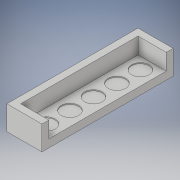
# Autodesk Inventor part: conteneur-boues
Saved by Autodesk Inventor 2019 (Build 230136000, 136)
## iProperties
Created: 2020-02-15
Part Number: conteneur-boues
Material: Generic
Document SubType Name: Modeling
Designer: franc
Density: 1 g/cm^3
Appearance: Default
Author: franc
Autodesk Inventor part; units mm, degrees
ref_plane "YZ Plane" through (0, 0, 0) normal (1, 0, 0) x (0, 1, 0)
ref_plane "XZ Plane" through (0, 0, 0) normal (0, 1, 0) x (-1, 0, 0)
ref_plane "XY Plane" through (0, 0, 0) normal (0, 0, 1) x (1, 0, 0)
sketch "Esquisse1" plane through (0, 0, 0) normal (0, 1, 0) x (-1, 0, 0)
  line L0 (56.6857, 276.3714) -> (-55.3143, 276.3714)
  line L1 (-55.3143, 276.3714) -> (-55.3143, -142.6286)
  line L2 (-55.3143, -142.6286) -> (56.6857, -142.6286)
  line L3 (56.6857, -142.6286) -> (56.6857, 276.3714)
  point P0 (0, 0)
  dimension "d0" = 112
  dimension "d1" = 419
  constraints: 8 end point, 2 parallel, 1 horizontal, 1 perpendicular
  measures "d0" distance of L1.end L2.end
  measures "d1" distance of L2.end L0.start
extrude "Extrusion1" add sketch "Esquisse1" along normal blind 22
sketch "Esquisse2" plane through (0, 22, 0) normal (0, 1, 0) x (1, 0, 0)
  line L0 (-56.6857, 142.6286) -> (-56.6857, -276.3714) projected
  line L1 (55.3143, -276.3714) -> (55.3143, 142.6286) projected
  line L2 (-56.6857, -276.3714) -> (55.3143, -276.3714)
  line L3 (55.3143, -276.3714) -> (55.3143, -254.3714)
  line L4 (55.3143, -254.3714) -> (-56.6857, -254.3714)
  line L5 (-56.6857, -254.3714) -> (-56.6857, -276.3714)
  line L6 (55.3143, 142.6286) -> (-56.6857, 142.6286) projected
  line L7 (-56.6857, 142.6286) -> (55.3143, 142.6286)
  line L8 (55.3143, 142.6286) -> (55.3143, 120.6286)
  line L9 (55.3143, 120.6286) -> (-56.6857, 120.6286)
  line L10 (-56.6857, 120.6286) -> (-56.6857, 142.6286)
  line L11 (-56.6857, -254.3714) -> (-34.6857, -254.3714)
  line L12 (-34.6857, -254.3714) -> (-34.6857, 120.6286)
  line L13 (-34.6857, 120.6286) -> (-56.6857, 120.6286)
  line L14 (-56.6857, 120.6286) -> (-56.6857, -254.3714)
  point P0 (0, 0)
  dimension "d4" = 22
  dimension "d5" = 22
  dimension "d6" = 22
  constraints: 24 end point, 6 parallel, 3 horizontal, 3 perpendicular, 3 point on line
  measures "d4" distance between parallel lines of L2 L4
  measures "d5" distance between parallel lines of L0 L12
  measures "d6" distance between parallel lines of L6 L9
extrude "Extrusion2" add sketch "Esquisse2" along normal blind 55 contours L6 L1 L9 L0 | L9 L12 L4 L0 | L4 L1 L2 L0
sketch "Esquisse3" plane through (0, 22, 0) normal (0, 1, 0) x (1, 0, 0)
  line L0 (-34.6857, 120.6286) -> (-34.6857, -254.3714) projected
  line L1 (-34.6857, 120.6286) -> (55.3143, 120.6286) projected
  line L2 (-34.6857, -254.3714) -> (55.3143, -254.3714)
  line L3 (55.3143, -254.3714) -> (55.3143, 120.6286)
  line L4 (55.3143, 120.6286) -> (-34.6857, 120.6286)
  line L5 (-34.6857, 120.6286) -> (-34.6857, -254.3714)
  circle A0 centre (10.3143, 83.1286) radius 28
  circle A1 centre (10.3143, 8.1286) radius 28
  circle A2 centre (10.3143, -66.8714) radius 28
  circle A3 centre (10.3143, -141.8714) radius 28
  circle A4 centre (10.3143, -216.8714) radius 28
  point P0 (0, 0)
  dimension "d9" = 37.5
  dimension "d10" = 45
  dimension "d11" = 56
  dimension "d12" = 75
  dimension "d13" = 56
  dimension "d14" = 45
  dimension "d15" = 56
  dimension "d16" = 45
  dimension "d17" = 75
  dimension "d18" = 56
  dimension "d19" = 45
  dimension "d20" = 75
  dimension "d21" = 45
  dimension "d22" = 75
  dimension "d23" = 56
  constraints: 8 end point, 5 centre point, 2 parallel, 1 horizontal, 1 perpendicular
  measures "d9" distance from line of L1 A0.centre
  measures "d10" distance from line of L3 A0.centre
  measures "d11" diameter of A0
  measures "d12" distance of A0.centre A1.centre
  measures "d13" diameter of A1
  measures "d14" distance from line of L3 A1.centre
  measures "d15" diameter of A2
  measures "d16" distance from line of L3 A2.centre
  measures "d17" distance of A1.centre A2.centre
  measures "d18" diameter of A3
  measures "d19" distance from line of L3 A3.centre
  measures "d20" distance of A2.centre A3.centre
  measures "d21" distance from line of L3 A4.centre
  measures "d22" distance of A3.centre A4.centre
  measures "d23" diameter of A4
extrude "Extrusion3" add sketch "Esquisse3" along normal blind 3
